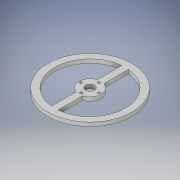
# Autodesk Inventor part: AcrylicFlywheel3
Saved by Autodesk Inventor 2018 (Build 220112000, 112)
## iProperties
Created: 2019-06-24
Part Number: AcrylicFlywheel3
Material: Generic
Document SubType Name: Modeling
Designer: anirudh
Density: 1 g/cm^3
Appearance: Default
Author: anirudh
Autodesk Inventor part; units mm, degrees
ref_plane "YZ Plane" through (0, 0, 0) normal (1, 0, 0) x (0, 1, 0)
ref_plane "XZ Plane" through (0, 0, 0) normal (0, 1, 0) x (-1, 0, 0)
ref_plane "XY Plane" through (0, 0, 0) normal (0, 0, 1) x (1, 0, 0)
sketch "Sketch1" plane through (0, 0, 0) normal (0, 1, 0) x (-1, 0, 0)
  circle A0 centre (0, 0) radius 63.5
  circle A1 centre (0, 0) radius 6.35
  circle A2 centre (-12.7, 0) radius 1.75
  circle A3 centre (0, -12.7) radius 1.75
  circle A4 centre (12.7, 0) radius 1.75
  circle A5 centre (0, 12.7) radius 1.75
  dimension "d8" = 3.5
  dimension "d9" = 3.5
  dimension "d10" = 3.5
  dimension "d11" = 3.5
  constraints: 6 centre point, 2 coincident
  measures "d8" diameter of A2
  measures "d9" diameter of A3
  measures "d10" diameter of A4
  measures "d11" diameter of A5
extrude "Extrusion1" add sketch "Sketch1" along normal blind 5.588
sketch "Sketch2" plane through (0, 5.588, 0) normal (0, 1, 0) x (1, 0, 0)
  circle A0 centre (0, 0) radius 63.5 projected
  line L0 (-4.7625, 37.8012) -> (-4.7625, 15.1438)
  line L1 (-4.7625, -15.1438) -> (-4.7625, -37.8012)
  line L2 (4.7625, 37.8012) -> (4.7625, 15.1438)
  line L3 (4.7625, -15.1438) -> (4.7625, -37.8012)
  arc A1 (-4.7625, 15.1438) -> (-4.7625, -15.1438) centre (0, 0) ccw
  arc A2 (4.7625, -15.1438) -> (4.7625, 15.1438) centre (0, 0) ccw
  arc A3 (-4.7625, 50.5763) -> (-4.7625, -50.5763) centre (0, 0) ccw
  arc A4 (4.7625, -50.5763) -> (4.7625, 50.5763) centre (0, 0) ccw
  line L4 (-4.7625, 50.5763) -> (-4.7625, 15.1438)
  line L5 (-4.7625, -15.1438) -> (-4.7625, -50.5763)
  line L6 (4.7625, -50.5763) -> (4.7625, -15.1438)
  line L7 (4.7625, 15.1438) -> (4.7625, 50.5763)
  constraints: 16 end point, 8 point on circle, 4 centre point, 4 vertical, 1 coincident
extrude "Extrusion3" cut sketch "Sketch2" against normal blind 25.4 contours L0 A1 L1 L5 A3 L4 | L7 A4 L6 L3 A2 L2
sketch "Sketch3" plane through (0, 5.588, 0) normal (0, 1, 0) x (1, 0, 0)
  circle A0 centre (0, 0) radius 63.5
  circle A1 centre (0, 0) radius 60.325
  dimension "d24" = 120.65
  constraints: 2 centre point, 2 coincident
  measures "d24" diameter of A1
extrude "Extrusion4" cut sketch "Sketch3" against normal blind 25.4
body "Solid1"
